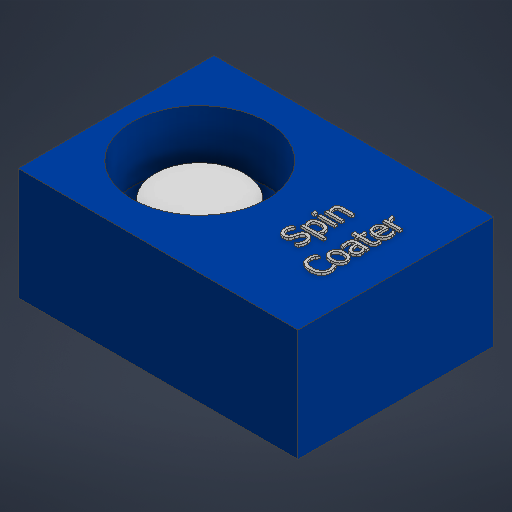
# Autodesk Inventor part: SpinCoater
Saved by Autodesk Inventor 2025.1 (Build 291241000, 241)
## iProperties
Created: 2024-10-04
Part Number: SpinCoater
Material: Generic
Document SubType Name: Modeling
Designer: jerem
Density: 1 g/cm^3
Appearance: Default
Author: jerem
Autodesk Inventor part; units mm, degrees
ref_plane "YZ Plane" through (0, 0, 0) normal (1, 0, 0) x (0, 1, 0)
ref_plane "XZ Plane" through (0, 0, 0) normal (0, 1, 0) x (-1, 0, 0)
ref_plane "XY Plane" through (0, 0, 0) normal (0, 0, 1) x (1, 0, 0)
sketch "Sketch1" plane through (0, 0, 0) normal (0, 1, 0) x (-1, 0, 0)
  line L0 (-125, -87.5) -> (125, -87.5)
  line L1 (125, -87.5) -> (125, 87.5)
  line L2 (125, 87.5) -> (-125, 87.5)
  line L3 (-125, 87.5) -> (-125, -87.5)
  line L4 (-125, -87.5) -> (125, 87.5) construction
  line L5 (125, -87.5) -> (-125, 87.5) construction
  circle A0 centre (49.9995, 0.22) radius 60
  circle A1 centre (49.9995, 0.22) radius 40
  line L6 (37.2995, -12.48) -> (62.6995, -12.48)
  line L7 (62.6995, -12.48) -> (62.6995, 12.92)
  line L8 (62.6995, 12.92) -> (37.2995, 12.92)
  line L9 (37.2995, 12.92) -> (37.2995, -12.48)
  line L10 (37.2995, -12.48) -> (62.6995, 12.92) construction
  line L11 (62.6995, -12.48) -> (37.2995, 12.92) construction
  line L12 (67.0408, -12.5) -> (92.0408, -12.5)
  line L13 (92.0408, -12.5) -> (92.0408, 12.5)
  line L14 (92.0408, 12.5) -> (67.0408, 12.5)
  line L15 (67.0408, 12.5) -> (67.0408, -12.5)
  line L16 (67.0408, -12.5) -> (92.0408, 12.5) construction
  line L17 (92.0408, -12.5) -> (67.0408, 12.5) construction
  line L18 (69.9864, -9.5545) -> (89.0953, -9.5545)
  line L19 (89.0953, -9.5545) -> (89.0953, 9.5545)
  line L20 (89.0953, 9.5545) -> (69.9864, 9.5545)
  line L21 (69.9864, 9.5545) -> (69.9864, -9.5545)
  line L22 (69.9864, -9.5545) -> (89.0953, 9.5545) construction
  line L23 (89.0953, -9.5545) -> (69.9864, 9.5545) construction
  line L24 (77.0408, -2.5) -> (82.0408, -2.5)
  line L25 (82.0408, -2.5) -> (82.0408, 2.5)
  line L26 (82.0408, 2.5) -> (77.0408, 2.5)
  line L27 (77.0408, 2.5) -> (77.0408, -2.5)
  line L28 (77.0408, -2.5) -> (82.0408, 2.5) construction
  line L29 (82.0408, -2.5) -> (77.0408, 2.5) construction
  line L30 (82.0408, 7.5) -> (87.0408, 7.5)
  line L31 (87.0408, 7.5) -> (87.0408, 2.5)
  line L32 (87.0408, 2.5) -> (82.0408, 2.5)
  line L33 (82.0408, 2.5) -> (82.0408, 7.5)
  line L34 (82.0408, 7.5) -> (87.0408, 2.5) construction
  line L35 (87.0408, 7.5) -> (82.0408, 2.5) construction
  line L36 (72.0408, -7.5) -> (77.0408, -7.5)
  line L37 (77.0408, -7.5) -> (77.0408, -2.5)
  line L38 (77.0408, -2.5) -> (72.0408, -2.5)
  line L39 (72.0408, -2.5) -> (72.0408, -7.5)
  line L40 (72.0408, -7.5) -> (77.0408, -2.5) construction
  line L41 (77.0408, -7.5) -> (72.0408, -2.5) construction
  line L42 (77.0408, 2.5) -> (72.0408, 2.5)
  line L43 (72.0408, 2.5) -> (72.0408, -2.5)
  line L44 (82.0408, -2.5) -> (87.0408, -2.5)
  line L45 (87.0408, -2.5) -> (87.0408, -7.5)
  line L46 (87.0408, -7.5) -> (82.0408, -7.5)
  line L47 (82.0408, -7.5) -> (82.0408, -2.5)
  line L48 (87.0408, -2.5) -> (82.0408, -2.5)
  line L49 (47.7195, 27.2613) -> (47.7195, 22.2613)
  line L50 (47.7195, 27.2613) -> (52.7195, 27.2613)
  line L51 (47.7195, 22.2613) -> (52.7195, 22.2613)
  line L52 (47.7195, 32.2613) -> (47.7195, 27.2613)
  line L53 (52.7195, 32.2613) -> (47.7195, 32.2613)
  line L54 (52.7195, 27.2613) -> (52.7195, 32.2613)
  line L55 (52.7195, 27.2613) -> (47.7195, 32.2613) construction
  line L56 (52.7195, 32.2613) -> (52.7195, 37.2613)
  line L57 (52.7195, 37.2613) -> (52.7195, 32.2613)
  line L58 (40.665, 20.2068) -> (59.774, 20.2068)
  line L59 (59.774, 20.2068) -> (59.774, 39.3158)
  line L60 (59.774, 39.3158) -> (40.665, 39.3158)
  line L61 (37.7195, 17.2613) -> (62.7195, 17.2613)
  line L62 (59.774, 39.3158) -> (40.665, 20.2068) construction
  line L63 (59.774, 20.2068) -> (40.665, 39.3158) construction
  line L64 (62.7195, 17.2613) -> (62.7195, 42.2613)
  line L65 (62.7195, 42.2613) -> (37.7195, 42.2613)
  line L66 (62.7195, 17.2613) -> (37.7195, 42.2613) construction
  line L67 (62.7195, 42.2613) -> (37.7195, 17.2613) construction
  line L68 (37.7195, 42.2613) -> (37.7195, 17.2613)
  line L69 (40.665, 39.3158) -> (40.665, 20.2068)
  line L70 (57.7195, 27.2613) -> (52.7195, 27.2613)
  line L71 (57.7195, 27.2613) -> (52.7195, 22.2613) construction
  line L72 (57.7195, 22.2613) -> (57.7195, 27.2613)
  line L73 (52.7195, 22.2613) -> (57.7195, 22.2613)
  line L74 (52.7195, 27.2613) -> (52.7195, 22.2613)
  line L75 (57.7195, 22.2613) -> (52.7195, 27.2613) construction
  line L76 (52.7195, 37.2613) -> (57.7195, 37.2613)
  line L77 (52.7195, 32.2613) -> (47.7195, 27.2613) construction
  line L78 (57.7195, 32.2613) -> (52.7195, 32.2613)
  line L79 (57.7195, 37.2613) -> (57.7195, 32.2613)
  line L80 (62.6995, 12.92) -> (37.2995, 12.92)
  line L81 (47.7195, 32.2613) -> (42.7195, 32.2613)
  line L82 (42.7195, 32.2613) -> (47.7195, 37.2613) construction
  line L83 (42.7195, 32.2613) -> (42.7195, 37.2613)
  line L84 (42.7195, 37.2613) -> (47.7195, 37.2613)
  line L85 (42.7195, 37.2613) -> (47.7195, 32.2613) construction
  line L86 (47.7195, 37.2613) -> (47.7195, 32.2613)
  line L87 (22.9582, -2.06) -> (27.9582, -2.06)
  line L88 (22.9582, -2.06) -> (22.9582, 2.94)
  line L89 (27.9582, -2.06) -> (27.9582, 2.94)
  line L90 (17.9582, -2.06) -> (22.9582, -2.06)
  line L91 (17.9582, 2.94) -> (17.9582, -2.06)
  line L92 (22.9582, 2.94) -> (17.9582, 2.94)
  line L93 (22.9582, 2.94) -> (17.9582, -2.06) construction
  line L94 (17.9582, 2.94) -> (12.9582, 2.94)
  line L95 (12.9582, 2.94) -> (17.9582, 2.94)
  line L96 (30.0127, -9.1145) -> (30.0127, 9.9944)
  line L97 (30.0127, 9.9944) -> (10.9037, 9.9944)
  line L98 (10.9037, 9.9944) -> (10.9037, -9.1145)
  line L99 (32.9582, -12.06) -> (32.9582, 12.94)
  line L100 (10.9037, 9.9944) -> (30.0127, -9.1145) construction
  line L101 (30.0127, 9.9944) -> (10.9037, -9.1145) construction
  line L102 (32.9582, 12.94) -> (7.9582, 12.94)
  line L103 (7.9582, 12.94) -> (7.9582, -12.06)
  line L104 (32.9582, 12.94) -> (7.9582, -12.06) construction
  line L105 (7.9582, 12.94) -> (32.9582, -12.06) construction
  line L106 (7.9582, -12.06) -> (32.9582, -12.06)
  line L107 (10.9037, -9.1145) -> (30.0127, -9.1145)
  line L108 (22.9582, 7.94) -> (22.9582, 2.94)
  line L109 (22.9582, 7.94) -> (27.9582, 2.94) construction
  line L110 (27.9582, 7.94) -> (22.9582, 7.94)
  line L111 (27.9582, 2.94) -> (27.9582, 7.94)
  line L112 (22.9582, 2.94) -> (27.9582, 2.94)
  line L113 (27.9582, 7.94) -> (22.9582, 2.94) construction
  line L114 (12.9582, 2.94) -> (12.9582, 7.94)
  line L115 (17.9582, 2.94) -> (22.9582, -2.06) construction
  line L116 (17.9582, 7.94) -> (17.9582, 2.94)
  line L117 (12.9582, 7.94) -> (17.9582, 7.94)
  line L118 (37.2995, 12.92) -> (37.2995, -12.48)
  line L119 (17.9582, -2.06) -> (17.9582, -7.06)
  line L120 (17.9582, -7.06) -> (12.9582, -2.06) construction
  line L121 (17.9582, -7.06) -> (12.9582, -7.06)
  line L122 (12.9582, -7.06) -> (12.9582, -2.06)
  line L123 (12.9582, -7.06) -> (17.9582, -2.06) construction
  line L124 (12.9582, -2.06) -> (17.9582, -2.06)
  line L125 (52.2795, -26.8213) -> (52.2795, -21.8213)
  line L126 (52.2795, -26.8213) -> (47.2795, -26.8213)
  line L127 (52.2795, -21.8213) -> (47.2795, -21.8213)
  line L128 (52.2795, -31.8213) -> (52.2795, -26.8213)
  line L129 (47.2795, -31.8213) -> (52.2795, -31.8213)
  line L130 (47.2795, -26.8213) -> (47.2795, -31.8213)
  line L131 (47.2795, -26.8213) -> (52.2795, -31.8213) construction
  line L132 (47.2795, -31.8213) -> (47.2795, -36.8213)
  line L133 (47.2795, -36.8213) -> (47.2795, -31.8213)
  line L134 (59.334, -19.7669) -> (40.2251, -19.7669)
  line L135 (40.2251, -19.7669) -> (40.2251, -38.8758)
  line L136 (40.2251, -38.8758) -> (59.334, -38.8758)
  line L137 (62.2795, -16.8213) -> (37.2795, -16.8213)
  line L138 (40.2251, -38.8758) -> (59.334, -19.7669) construction
  line L139 (40.2251, -19.7669) -> (59.334, -38.8758) construction
  line L140 (37.2795, -16.8213) -> (37.2795, -41.8213)
  line L141 (37.2795, -41.8213) -> (62.2795, -41.8213)
  line L142 (37.2795, -16.8213) -> (62.2795, -41.8213) construction
  line L143 (37.2795, -41.8213) -> (62.2795, -16.8213) construction
  line L144 (62.2795, -41.8213) -> (62.2795, -16.8213)
  line L145 (59.334, -38.8758) -> (59.334, -19.7669)
  line L146 (42.2795, -26.8213) -> (47.2795, -26.8213)
  line L147 (42.2795, -26.8213) -> (47.2795, -21.8213) construction
  line L148 (42.2795, -21.8213) -> (42.2795, -26.8213)
  line L149 (47.2795, -21.8213) -> (42.2795, -21.8213)
  line L150 (47.2795, -26.8213) -> (47.2795, -21.8213)
  line L151 (42.2795, -21.8213) -> (47.2795, -26.8213) construction
  line L152 (47.2795, -36.8213) -> (42.2795, -36.8213)
  line L153 (47.2795, -31.8213) -> (52.2795, -26.8213) construction
  line L154 (42.2795, -31.8213) -> (47.2795, -31.8213)
  line L155 (42.2795, -36.8213) -> (42.2795, -31.8213)
  line L156 (37.2995, -12.48) -> (62.6995, -12.48)
  line L157 (52.2795, -31.8213) -> (57.2795, -31.8213)
  line L158 (57.2795, -31.8213) -> (52.2795, -36.8213) construction
  line L159 (57.2795, -31.8213) -> (57.2795, -36.8213)
  line L160 (57.2795, -36.8213) -> (52.2795, -36.8213)
  line L161 (57.2795, -36.8213) -> (52.2795, -31.8213) construction
  line L162 (52.2795, -36.8213) -> (52.2795, -31.8213)
  point P0 (0, 0)
  point P1 (79.5408, 0)
  point P2 (84.5408, 5)
  point P3 (74.5408, -5)
  point P4 (50.2195, 29.7613)
  point P5 (45.2195, 34.7613)
  point P6 (55.2195, 24.7613)
  point P7 (20.4582, 0.44)
  point P8 (15.4582, -4.56)
  point P9 (25.4582, 5.44)
  point P10 (49.7795, -29.3213)
  point P11 (54.7795, -34.3213)
  point P12 (44.7795, -24.3213)
  dimension "d0" = 175
  dimension "d1" = 250
  dimension "d6" = 120
  dimension "d7" = 80
  dimension "d8" = 50
  dimension "d13" = 25.4
  dimension "d14" = 25.4
  dimension "d15" = 25
  dimension "d16" = 25
  dimension "d17" = 5
  dimension "d18" = 5
  dimension "d19" = 5
  dimension "d20" = 5
  dimension "d21" = 5
  dimension "d22" = 5
  dimension "d23" = 5
  dimension "d26" = 360
  constraints: 326 end point, 24 point on line, 14 midpoint, 14 parallel, 12 perpendicular, 8 horizontal, 2 centre point, 1 coincident, 269 other
  measures "d0" distance of L0.end L1.end
  measures "d1" distance of L1.end L2.end
  measures "d6" diameter of A0
  measures "d7" diameter of A1
  measures "d8" distance of point (0, 0) A0.centre
  measures "d13" distance of L8.end L7.end
  measures "d14" distance of L7.end L6.end
  measures "d15" distance of L14.end L13.end
  measures "d16" distance of L13.end L12.end
  measures "d17" distance of L26.end L25.end
  measures "d18" distance of L25.end L24.end
  measures "d19" distance of L31.end L32.end
  measures "d20" distance of L30.end L31.end
  measures "d21" distance of L38.end L37.end
  measures "d22" distance of L37.end L36.end
  measures "d23" distance of L44.end L45.end
extrude "Extrusion1" add sketch "Sketch1" along normal blind 100 contours L3 L2 L1 L0 | A0 | A1 L19 | A1 L19 L20 L14 L13 L12 L18 | L19 A1 L18 L21 L20 | A1 L20 L19 | L19 L18 A1 | L20 L21 L18 A1 L12 L15 L14 | L14 L15 L12 A1 L144 L137 L140 L106 L99 L102 L68 L61 L64 | L64 L61 L68 A1 L69 L58 L59 | A1 L59 L60 L69 L68 L65 L64 | L144 L141 L140 A1 L135 L136 L145 | A1 L145 L134 L135 L140 L137 L144 | L59 L58 L69 A1 L60 | A1 L60 L59 | L145 L136 A1 | A1 L136 L135 L134 L145 | L60 A1 | A1 L136 | A1 L69 L60 | L136 L135 A1 | L102 L99 L106 A1 L107 L96 L97 | A1 L97 L98 L107 L106 L103 L102 | L97 L96 L107 A1 L98 | A1 L98 L97 | L107 L98 A1 | L98 A1 | L9 L8 L7 L6 | L27 L26 L25 L24 | L38 L43 L42 L27 | L33 L30 L31 L32 | L44 L45 L46 L47 | L37 L36 L39 L38 | L50 L74 L51 L49 | L52 L53 L54 L50 | L81 L83 L84 L86 | L56 L76 L79 L78 | L70 L72 L73 L74 | L88 L112 L89 L87 | L90 L91 L92 L88 | L119 L121 L122 L124 | L94 L114 L117 L116 | L108 L110 L111 L112 | L126 L150 L127 L125 | L128 L129 L130 L126 | L157 L159 L160 L162 | L132 L152 L155 L154 | L146 L148 L149 L150
extrude "Extrusion3" cut sketch "Sketch1" against normal blind 50 from surface at 100 contours A0 | A1 L19 | A1 L19 L20 L14 L13 L12 L18 | L19 A1 L18 L21 L20 | A1 L20 L19 | L19 L18 A1 | L20 L21 L18 A1 L12 L15 L14 | L14 L15 L12 A1 L144 L137 L140 L106 L99 L102 L68 L61 L64 | L64 L61 L68 A1 L69 L58 L59 | A1 L59 L60 L69 L68 L65 L64 | L144 L141 L140 A1 L135 L136 L145 | A1 L145 L134 L135 L140 L137 L144 | L59 L58 L69 A1 L60 | A1 L60 L59 | L145 L136 A1 | A1 L136 L135 L134 L145 | L60 A1 | A1 L136 | A1 L69 L60 | L136 L135 A1 | L102 L99 L106 A1 L107 L96 L97 | A1 L97 L98 L107 L106 L103 L102 | L97 L96 L107 A1 L98 | A1 L98 L97 | L107 L98 A1 | L98 A1 | L9 L8 L7 L6 | L27 L26 L25 L24 | L38 L43 L42 L27 | L33 L30 L31 L32 | L44 L45 L46 L47 | L37 L36 L39 L38 | L50 L74 L51 L49 | L52 L53 L54 L50 | L81 L83 L84 L86 | L56 L76 L79 L78 | L70 L72 L73 L74 | L88 L112 L89 L87 | L90 L91 L92 L88 | L119 L121 L122 L124 | L94 L114 L117 L116 | L108 L110 L111 L112 | L126 L150 L127 L125 | L128 L129 L130 L126 | L157 L159 L160 L162 | L132 L152 L155 L154 | L146 L148 L149 L150
extrude "Extrusion4" add sketch "Sketch1" along normal blind 20 from surface at 50 contours A1 L19 | L19 A1 L18 L21 L20 | L20 L21 L18 A1 L12 L15 L14 | L14 L15 L12 A1 L144 L137 L140 L106 L99 L102 L68 L61 L64 | L64 L61 L68 A1 L69 L58 L59 | A1 L145 L134 L135 L140 L137 L144 | L59 L58 L69 A1 L60 | A1 L136 L135 L134 L145 | L60 A1 | A1 L136 | L102 L99 L106 A1 L107 L96 L97 | L97 L96 L107 A1 L98 | L98 A1 | L9 L8 L7 L6 | L27 L26 L25 L24 | L38 L43 L42 L27 | L33 L30 L31 L32 | L44 L45 L46 L47 | L37 L36 L39 L38 | L50 L74 L51 L49 | L52 L53 L54 L50 | L81 L83 L84 L86 | L56 L76 L79 L78 | L70 L72 L73 L74 | L88 L112 L89 L87 | L90 L91 L92 L88 | L119 L121 L122 L124 | L94 L114 L117 L116 | L108 L110 L111 L112 | L126 L150 L127 L125 | L128 L129 L130 L126 | L157 L159 L160 L162 | L132 L152 L155 L154 | L146 L148 L149 L150
sketch "Sketch3" plane through (0, 100, 0) normal (0, 1, 0) x (1, 0, 0)
  line L0 (29.7079, -63.6331) -> (29.7079, 66.3057) construction
  line L1 (29.7079, 66.3057) -> (108.1288, 66.3057) construction
  line L2 (108.1288, 66.3057) -> (108.1288, -63.6331) construction
  line L3 (108.1288, -63.6331) -> (29.7079, -63.6331) construction
  spline S0 degree 2 poles (62.7777, -17.1321) (62.7777, -19.3039) (61.8701, -22.3509) (61.2218, -23.6961) knots 0 0 0 1 2 2 2
  line L4 (61.2218, -23.6961) -> (57.8831, -23.6961)
  line L5 (57.8831, -23.6961) -> (57.8831, -23.5016)
  spline S1 degree 2 poles (57.8831, -23.5016) (59.1148, -22.1888) (60.4763, -18.8663) (60.4763, -17.3266) knots 0 0 0 1 2 2 2
  spline S2 degree 2 poles (60.4763, -17.3266) (60.4763, -15.1224) (58.6448, -12.8695) (57.1375, -12.8695) knots 0 0 0 1 2 2 2
  spline S3 degree 2 poles (57.1375, -12.8695) (55.9382, -12.8695) (54.4471, -14.0527) (54.0743, -15.3331) knots 0 0 0 1 2 2 2
  spline S4 degree 2 poles (54.0743, -15.3331) (53.815, -16.2569) (53.4584, -17.7966) (53.1667, -18.9473) knots 0 0 0 1 2 2 2
  spline S5 degree 2 poles (53.1667, -18.9473) (52.8912, -19.9846) (52.0646, -21.6216) (51.4001, -22.2537) knots 0 0 0 1 2 2 2
  spline S6 degree 2 poles (51.4001, -22.2537) (50.7356, -22.8695) (48.9528, -23.5502) (47.7858, -23.5502) knots 0 0 0 1 2 2 2
  spline S7 degree 2 poles (47.7858, -23.5502) (45.3547, -23.5502) (42.0646, -19.7577) (42.0646, -16.8242) knots 0 0 0 1 2 2 2
  spline S8 degree 2 poles (42.0646, -16.8242) (42.0646, -15.1386) (42.7291, -12.1564) (43.3612, -10.876) knots 0 0 0 1 2 2 2
  line L6 (43.3612, -10.876) -> (46.5379, -10.876)
  line L7 (46.5379, -10.876) -> (46.5379, -11.0705)
  spline S9 degree 2 poles (46.5379, -11.0705) (45.6627, -12.0267) (44.3661, -15.0089) (44.3661, -16.6459) knots 0 0 0 1 2 2 2
  spline S10 degree 2 poles (44.3661, -16.6459) (44.3661, -18.4935) (46.1003, -20.7788) (47.5103, -20.7788) knots 0 0 0 1 2 2 2
  spline S11 degree 2 poles (47.5103, -20.7788) (48.7745, -20.7788) (50.2818, -19.4336) (50.6221, -18.1694) knots 0 0 0 1 2 2 2
  spline S12 degree 2 poles (50.6221, -18.1694) (50.849, -17.3266) (51.4325, -14.8793) (51.6756, -14.0689) knots 0 0 0 1 2 2 2
  spline S13 degree 2 poles (51.6756, -14.0689) (52.3077, -12.0105) (54.8523, -10.0981) (56.7161, -10.0981) knots 0 0 0 1 2 2 2
  spline S14 degree 2 poles (56.7161, -10.0981) (57.8993, -10.0981) (60.1683, -11.0543) (60.9625, -11.9133) knots 0 0 0 1 2 2 2
  spline S15 degree 2 poles (60.9625, -11.9133) (61.8377, -12.8695) (62.7777, -15.3007) (62.7777, -17.1321) knots 0 0 0 1 2 2 2
  spline S16 degree 2 poles (54.5119, 4.9911) (58.2721, 4.9911) (62.7129, 1.4092) (62.7129, -1.3298) knots 0 0 0 1 2 2 2
  spline S17 degree 2 poles (62.7129, -1.3298) (62.7129, -2.4481) (62.1943, -4.1661) (61.6594, -5.0575) knots 0 0 0 1 2 2 2
  line L8 (61.6594, -5.0575) -> (67.9479, -5.0575)
  line L9 (67.9479, -5.0575) -> (67.9479, -7.5859)
  line L10 (67.9479, -7.5859) -> (47.4131, -7.5859)
  line L11 (47.4131, -7.5859) -> (47.4131, -5.0575)
  line L12 (47.4131, -5.0575) -> (48.9852, -5.0575)
  spline S18 degree 2 poles (48.9852, -5.0575) (48.1262, -4.1175) (46.9917, -1.816) (46.9917, -0.4708) knots 0 0 0 1 2 2 2
  spline S19 degree 2 poles (46.9917, -0.4708) (46.9917, 2.1062) (51.0759, 4.9911) (54.5119, 4.9911) knots 0 0 0 1 2 2 2
  spline S20 degree 2 poles (54.8037, 2.3817) (52.2267, 2.3817) (49.3904, 0.7447) (49.3904, -1.0867) knots 0 0 0 1 2 2 2
  spline S21 degree 2 poles (49.3904, -1.0867) (49.3904, -2.1564) (50.3466, -4.1661) (51.0922, -5.0575) knots 0 0 0 1 2 2 2
  line L13 (51.0922, -5.0575) -> (59.6173, -5.0575)
  spline S22 degree 2 poles (59.6173, -5.0575) (60.0873, -4.0689) (60.4439, -2.6588) (60.4439, -1.7512) knots 0 0 0 1 2 2 2
  spline S23 degree 2 poles (60.4439, -1.7512) (60.4439, 0.2099) (57.5589, 2.3817) (54.8037, 2.3817) knots 0 0 0 1 2 2 2
  line L14 (62.4212, 10.1937) -> (62.4212, 7.6653)
  line L15 (62.4212, 7.6653) -> (47.4131, 7.6653)
  line L16 (47.4131, 7.6653) -> (47.4131, 10.1937)
  line L17 (47.4131, 10.1937) -> (62.4212, 10.1937)
  line L18 (44.9171, 10.372) -> (44.9171, 7.5032)
  line L19 (44.9171, 7.5032) -> (42.2915, 7.5032)
  line L20 (42.2915, 7.5032) -> (42.2915, 10.372)
  line L21 (42.2915, 10.372) -> (44.9171, 10.372)
  line L22 (62.4212, 25.688) -> (62.4212, 23.1596)
  line L23 (62.4212, 23.1596) -> (53.8636, 23.1596)
  spline S24 degree 2 poles (53.8636, 23.1596) (52.8264, 23.1596) (51.0435, 22.9652) (50.5087, 22.6734) knots 0 0 0 1 2 2 2
  spline S25 degree 2 poles (50.5087, 22.6734) (49.9414, 22.3655) (49.3904, 21.2634) (49.3904, 20.3233) knots 0 0 0 1 2 2 2
  spline S26 degree 2 poles (49.3904, 20.3233) (49.3904, 19.3833) (50.3952, 17.3898) (51.2056, 16.4335) knots 0 0 0 1 2 2 2
  line L24 (51.2056, 16.4335) -> (62.4212, 16.4335)
  line L25 (62.4212, 16.4335) -> (62.4212, 13.9052)
  line L26 (62.4212, 13.9052) -> (47.4131, 13.9052)
  line L27 (47.4131, 13.9052) -> (47.4131, 16.4335)
  line L28 (47.4131, 16.4335) -> (49.0824, 16.4335)
  spline S27 degree 2 poles (49.0824, 16.4335) (48.0614, 17.5681) (46.9917, 19.7561) (46.9917, 20.9878) knots 0 0 0 1 2 2 2
  spline S28 degree 2 poles (46.9917, 20.9878) (46.9917, 23.1921) (49.909, 25.688) (52.6805, 25.688) knots 0 0 0 1 2 2 2
  line L29 (52.6805, 25.688) -> (62.4212, 25.688)
  spline S29 degree 2 poles (95.7072, -28.5665) (95.7072, -30.5113) (94.3944, -33.8015) (93.0816, -35.0008) knots 0 0 0 1 2 2 2
  spline S30 degree 2 poles (93.0816, -35.0008) (91.785, -36.2002) (87.8952, -37.513) (85.3668, -37.513) knots 0 0 0 1 2 2 2
  spline S31 degree 2 poles (85.3668, -37.513) (82.8547, -37.513) (79.127, -36.2326) (77.7493, -35.017) knots 0 0 0 1 2 2 2
  spline S32 degree 2 poles (77.7493, -35.017) (76.4041, -33.8177) (74.9941, -30.5438) (74.9941, -28.5178) knots 0 0 0 1 2 2 2
  spline S33 degree 2 poles (74.9941, -28.5178) (74.9941, -27.513) (75.2858, -25.7464) (75.5127, -25.0008) knots 0 0 0 1 2 2 2
  spline S34 degree 2 poles (75.5127, -25.0008) (75.7234, -24.3525) (76.3231, -23.0073) (76.6797, -22.3428) knots 0 0 0 1 2 2 2
  line L30 (76.6797, -22.3428) -> (79.8887, -22.3428)
  line L31 (79.8887, -22.3428) -> (79.8887, -22.5535)
  spline S35 degree 2 poles (79.8887, -22.5535) (79.5646, -22.9101) (78.657, -24.0122) (78.2194, -24.8063) knots 0 0 0 1 2 2 2
  spline S36 degree 2 poles (78.2194, -24.8063) (77.798, -25.5681) (77.2631, -27.3671) (77.2631, -28.534) knots 0 0 0 1 2 2 2
  spline S37 degree 2 poles (77.2631, -28.534) (77.2631, -29.8144) (78.3166, -32.0997) (79.3215, -32.9587) knots 0 0 0 1 2 2 2
  spline S38 degree 2 poles (79.3215, -32.9587) (80.3425, -33.8015) (83.4382, -34.7415) (85.3668, -34.7415) knots 0 0 0 1 2 2 2
  spline S39 degree 2 poles (85.3668, -34.7415) (87.4252, -34.7415) (90.3912, -33.7528) (91.4122, -32.8938) knots 0 0 0 1 2 2 2
  spline S40 degree 2 poles (91.4122, -32.8938) (92.4009, -32.0511) (93.4057, -29.7982) (93.4057, -28.534) knots 0 0 0 1 2 2 2
  spline S41 degree 2 poles (93.4057, -28.534) (93.4057, -27.3833) (92.8385, -25.4222) (92.4171, -24.6605) knots 0 0 0 1 2 2 2
  spline S42 degree 2 poles (92.4171, -24.6605) (91.9957, -23.9311) (91.1205, -22.8452) (90.8126, -22.5373) knots 0 0 0 1 2 2 2
  line L32 (90.8126, -22.5373) -> (90.8126, -22.3428)
  line L33 (90.8126, -22.3428) -> (93.9892, -22.3428)
  spline S43 degree 2 poles (93.9892, -22.3428) (94.2972, -23.0073) (94.8644, -24.1742) (95.1237, -25.0008) knots 0 0 0 1 2 2 2
  spline S44 degree 2 poles (95.1237, -25.0008) (95.4155, -25.876) (95.7072, -27.3671) (95.7072, -28.5665) knots 0 0 0 1 2 2 2
  spline S45 degree 2 poles (87.8466, -7.7237) (91.6391, -7.7237) (95.772, -11.3703) (95.772, -14.4173) knots 0 0 0 1 2 2 2
  spline S46 degree 2 poles (95.772, -14.4173) (95.772, -17.5454) (91.5095, -21.1272) (87.8466, -21.1272) knots 0 0 0 1 2 2 2
  spline S47 degree 2 poles (87.8466, -21.1272) (84.0865, -21.1272) (79.9211, -17.4319) (79.9211, -14.4173) knots 0 0 0 1 2 2 2
  spline S48 degree 2 poles (79.9211, -14.4173) (79.9211, -11.3703) (84.0703, -7.7237) (87.8466, -7.7237) knots 0 0 0 1 2 2 2
  spline S49 degree 2 poles (87.8466, -10.3331) (84.9292, -10.3331) (82.0929, -12.4562) (82.0929, -14.4173) knots 0 0 0 1 2 2 2
  spline S50 degree 2 poles (82.0929, -14.4173) (82.0929, -16.3784) (84.9292, -18.5178) (87.8466, -18.5178) knots 0 0 0 1 2 2 2
  spline S51 degree 2 poles (87.8466, -18.5178) (90.6829, -18.5178) (93.6002, -16.3784) (93.6002, -14.4173) knots 0 0 0 1 2 2 2
  spline S52 degree 2 poles (93.6002, -14.4173) (93.6002, -12.4725) (90.7315, -10.3331) (87.8466, -10.3331) knots 0 0 0 1 2 2 2
  spline S53 degree 2 poles (93.7623, 3.2326) (93.9892, 2.9246) (94.7996, 1.8874) (95.0427, 1.4011) knots 0 0 0 1 2 2 2
  spline S54 degree 2 poles (95.0427, 1.4011) (95.3993, 0.7366) (95.772, -0.5113) (95.772, -1.6459) knots 0 0 0 1 2 2 2
  spline S55 degree 2 poles (95.772, -1.6459) (95.772, -2.5697) (95.0751, -4.2391) (94.443, -4.8712) knots 0 0 0 1 2 2 2
  spline S56 degree 2 poles (94.443, -4.8712) (93.8271, -5.4708) (92.0119, -6.2002) (91.007, -6.2002) knots 0 0 0 1 2 2 2
  spline S57 degree 2 poles (91.007, -6.2002) (89.4511, -6.2002) (87.2469, -4.8874) (86.6148, -3.4611) knots 0 0 0 1 2 2 2
  spline S58 degree 2 poles (86.6148, -3.4611) (86.0314, -2.1969) (85.5938, 1.2391) (85.4803, 3.2326) knots 0 0 0 1 2 2 2
  line L34 (85.4803, 3.2326) -> (84.9941, 3.2326)
  spline S59 degree 2 poles (84.9941, 3.2326) (84.1189, 3.2326) (83.033, 2.6977) (82.725, 2.2115) knots 0 0 0 1 2 2 2
  spline S60 degree 2 poles (82.725, 2.2115) (82.4171, 1.7253) (82.2226, 0.3314) (82.2226, -0.4141) knots 0 0 0 1 2 2 2
  spline S61 degree 2 poles (82.2226, -0.4141) (82.2226, -1.2893) (82.7412, -3.6556) (83.2437, -4.8387) knots 0 0 0 1 2 2 2
  line L35 (83.2437, -4.8387) -> (83.2437, -4.9846)
  line L36 (83.2437, -4.9846) -> (80.6667, -4.9846)
  spline S62 degree 2 poles (80.6667, -4.9846) (80.4722, -4.2877) (79.986, -1.6783) (79.986, -0.3979) knots 0 0 0 1 2 2 2
  spline S63 degree 2 poles (79.986, -0.3979) (79.986, 1.158) (80.4722, 3.2812) (81.1043, 4.124) knots 0 0 0 1 2 2 2
  spline S64 degree 2 poles (81.1043, 4.124) (81.7202, 4.9506) (83.6813, 5.7609) (85.0913, 5.7609) knots 0 0 0 1 2 2 2
  line L37 (85.0913, 5.7609) -> (95.3506, 5.7609)
  line L38 (95.3506, 5.7609) -> (95.3506, 3.2326)
  line L39 (95.3506, 3.2326) -> (93.7623, 3.2326)
  line L40 (91.6553, 3.2326) -> (87.49, 3.2326)
  spline S65 degree 2 poles (87.49, 3.2326) (87.5711, 2.325) (87.8466, -0.4141) (88.1059, -1.2731) knots 0 0 0 1 2 2 2
  spline S66 degree 2 poles (88.1059, -1.2731) (88.4138, -2.278) (89.6942, -3.5908) (90.8288, -3.5908) knots 0 0 0 1 2 2 2
  spline S67 degree 2 poles (90.8288, -3.5908) (92.1254, -3.5908) (93.4382, -2.1321) (93.4382, -0.7383) knots 0 0 0 1 2 2 2
  spline S68 degree 2 poles (93.4382, -0.7383) (93.4382, 0.4449) (92.4171, 2.3898) (91.6553, 3.2326) knots 0 0 0 1 2 2 2
  spline S69 degree 2 poles (95.6424, 13.8485) (95.6424, 11.7901) (93.2923, 9.4724) (90.7477, 9.4724) knots 0 0 0 1 2 2 2
  line L41 (90.7477, 9.4724) -> (82.4333, 9.4724)
  line L42 (82.4333, 9.4724) -> (82.4333, 7.7707)
  line L43 (82.4333, 7.7707) -> (80.3425, 7.7707)
  line L44 (80.3425, 7.7707) -> (80.3425, 9.4724)
  line L45 (80.3425, 9.4724) -> (76.0314, 9.4724)
  line L46 (76.0314, 9.4724) -> (76.0314, 12.0008)
  line L47 (76.0314, 12.0008) -> (80.3425, 12.0008)
  line L48 (80.3425, 12.0008) -> (80.3425, 16.6523)
  line L49 (80.3425, 16.6523) -> (82.4333, 16.6523)
  line L50 (82.4333, 16.6523) -> (82.4333, 12.0008)
  line L51 (82.4333, 12.0008) -> (89.5808, 12.0008)
  spline S70 degree 2 poles (89.5808, 12.0008) (90.7153, 12.0008) (91.9633, 12.0818) (92.4981, 12.3574) knots 0 0 0 1 2 2 2
  spline S71 degree 2 poles (92.4981, 12.3574) (92.9681, 12.5843) (93.4382, 13.6053) (93.4382, 14.4805) knots 0 0 0 1 2 2 2
  spline S72 degree 2 poles (93.4382, 14.4805) (93.4382, 15.0964) (93.0654, 16.2472) (92.9519, 16.5065) knots 0 0 0 1 2 2 2
  line L52 (92.9519, 16.5065) -> (92.9519, 16.6523)
  line L53 (92.9519, 16.6523) -> (95.221, 16.6523)
  spline S73 degree 2 poles (95.221, 16.6523) (95.4155, 15.9392) (95.6424, 14.4805) (95.6424, 13.8485) knots 0 0 0 1 2 2 2
  spline S74 degree 2 poles (95.691, 25.0316) (95.691, 21.4335) (91.6553, 17.4789) (87.9276, 17.4789) knots 0 0 0 1 2 2 2
  spline S75 degree 2 poles (87.9276, 17.4789) (84.2647, 17.4789) (79.9211, 21.3201) (79.9211, 24.4157) knots 0 0 0 1 2 2 2
  spline S76 degree 2 poles (79.9211, 24.4157) (79.9211, 25.8096) (80.7315, 27.9652) (81.5905, 28.7593) knots 0 0 0 1 2 2 2
  spline S77 degree 2 poles (81.5905, 28.7593) (82.4495, 29.5697) (84.9292, 30.4287) (86.7283, 30.4287) knots 0 0 0 1 2 2 2
  line L54 (86.7283, 30.4287) -> (88.1059, 30.4287)
  line L55 (88.1059, 30.4287) -> (88.1059, 20.0397)
  spline S78 degree 2 poles (88.1059, 20.0397) (90.7153, 20.0397) (93.4868, 22.6653) (93.4868, 24.9992) knots 0 0 0 1 2 2 2
  spline S79 degree 2 poles (93.4868, 24.9992) (93.4868, 25.8258) (93.114, 27.4303) (92.8223, 28.0786) knots 0 0 0 1 2 2 2
  spline S80 degree 2 poles (92.8223, 28.0786) (92.4981, 28.7593) (91.9309, 29.6993) (91.6715, 30.0073) knots 0 0 0 1 2 2 2
  line L56 (91.6715, 30.0073) -> (91.6715, 30.1532)
  line L57 (91.6715, 30.1532) -> (94.4268, 30.1532)
  spline S81 degree 2 poles (94.4268, 30.1532) (94.6051, 29.7156) (95.1237, 28.3865) (95.2696, 27.8679) knots 0 0 0 1 2 2 2
  spline S82 degree 2 poles (95.2696, 27.8679) (95.4803, 27.1386) (95.691, 25.9392) (95.691, 25.0316) knots 0 0 0 1 2 2 2
  spline S83 degree 2 poles (86.1772, 27.9652) (85.1562, 27.9327) (83.6651, 27.5113) (83.1626, 27.1062) knots 0 0 0 1 2 2 2
  spline S84 degree 2 poles (83.1626, 27.1062) (82.5954, 26.6686) (81.9957, 25.2909) (81.9957, 24.2699) knots 0 0 0 1 2 2 2
  spline S85 degree 2 poles (81.9957, 24.2699) (81.9957, 23.265) (82.5954, 21.8549) (83.1788, 21.2715) knots 0 0 0 1 2 2 2
  spline S86 degree 2 poles (83.1788, 21.2715) (83.7785, 20.7042) (85.221, 20.1207) (86.1772, 20.0397) knots 0 0 0 1 2 2 2
  line L58 (86.1772, 20.0397) -> (86.1772, 27.9652)
  line L59 (83.0492, 40.9473) -> (83.0492, 40.8177)
  spline S87 degree 2 poles (83.0492, 40.8177) (82.9681, 40.5259) (82.9357, 39.8938) (82.9357, 39.4562) knots 0 0 0 1 2 2 2
  spline S88 degree 2 poles (82.9357, 39.4562) (82.9357, 38.4352) (83.8271, 36.4254) (84.7023, 35.5178) knots 0 0 0 1 2 2 2
  line L60 (84.7023, 35.5178) -> (95.3506, 35.5178)
  line L61 (95.3506, 35.5178) -> (95.3506, 32.9895)
  line L62 (95.3506, 32.9895) -> (80.3425, 32.9895)
  line L63 (80.3425, 32.9895) -> (80.3425, 35.5178)
  line L64 (80.3425, 35.5178) -> (82.5792, 35.5178)
  spline S89 degree 2 poles (82.5792, 35.5178) (81.3474, 36.8955) (80.3425, 38.9538) (80.3425, 39.9263) knots 0 0 0 1 2 2 2
  spline S90 degree 2 poles (80.3425, 39.9263) (80.3425, 40.3152) (80.375, 40.7042) (80.4236, 40.9473) knots 0 0 0 1 2 2 2
  line L65 (80.4236, 40.9473) -> (83.0492, 40.9473)
  point P0 (0, 0)
  constraints: 1 coincident, 2 other
extrude "Extrusion2" add sketch "Sketch3" along normal blind 2
body "Solid1"
